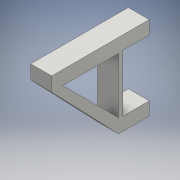
# Autodesk Inventor part: ServoSupport
Saved by Autodesk Inventor 2016 (Build 200138000, 138)
## iProperties
Created: 2016-04-17
Part Number: ServoSupport
Material: PC/ABS Plastic
Document SubType Name: Modeling
Designer: amenoni
Density: 0.357273 g/cm^3
Appearance: Smooth - White
Author: amenoni
Autodesk Inventor part; units mm, degrees
ref_plane "YZ Plane" through (0, 0, 0) normal (1, 0, 0) x (0, 1, 0)
ref_plane "XZ Plane" through (0, 0, 0) normal (0, 1, 0) x (-1, 0, 0)
ref_plane "XY Plane" through (0, 0, 0) normal (0, 0, 1) x (1, 0, 0)
sketch "Sketch1" plane through (0, 0, 0) normal (0, 1, 0) x (-1, 0, 0)
  line L0 (-7.5, -30) -> (7.5, -30)
  line L1 (7.5, -30) -> (7.5, 30)
  line L2 (7.5, 30) -> (-7.5, 30)
  line L3 (-7.5, 30) -> (-7.5, -30)
  line L4 (-7.5, -30) -> (7.5, 30) construction
  line L5 (7.5, -30) -> (-7.5, 30) construction
  point P0 (0, 0)
  dimension "d0" = 15
  dimension "d1" = 60
  constraints: 12 end point, 2 midpoint, 2 parallel, 1 horizontal, 1 perpendicular
  measures "d0" distance of L2.end L1.end
  measures "d1" distance of L1.end L0.end
extrude "Extrusion1" add sketch "Sketch1" along normal blind 3
sketch "Sketch2" plane through (0, 3, 0) normal (0, 1, 0) x (1, 0, 0)
  line L0 (-7.5, 30) -> (-7.5, -30) projected
  line L1 (7.5, 20.5) -> (-7.5, 20.5)
  line L2 (-7.5, 20.5) -> (-7.5, -20.5)
  line L3 (-7.5, -20.5) -> (7.5, -20.5)
  line L4 (7.5, -20.5) -> (7.5, 20.5)
  line L5 (7.5, 20.5) -> (-7.5, -20.5) construction
  line L6 (-7.5, 20.5) -> (7.5, -20.5) construction
  line L7 (7.5, -20.5) -> (-7.5, -20.5)
  line L8 (-7.5, -20.5) -> (-7.5, -30)
  line L9 (-7.5, -30) -> (7.5, -30)
  line L10 (7.5, -30) -> (7.5, -20.5)
  line L11 (7.5, 30) -> (-7.5, 30) projected
  line L12 (7.5, 20.5) -> (-7.5, 20.5)
  line L13 (-7.5, 20.5) -> (-7.5, 30)
  line L14 (-7.5, 30) -> (7.5, 30)
  line L15 (7.5, 30) -> (7.5, 20.5)
  point P0 (0, 0)
  dimension "d4" = 41
  constraints: 28 end point, 6 parallel, 3 horizontal, 3 perpendicular, 2 midpoint, 1 point on line
  measures "d4" distance of L2.end L1.end
extrude "Extrusion2" add sketch "Sketch2" along normal blind 19 contours L11 L15 L1 L0 | L3 L10 L9 L0
sketch "Sketch3" plane through (-7.5, 0, -30) normal (-1, 0, 0) x (0, 0, 1)
  line L0 (60, 0) -> (0, 0) projected
  line L1 (60, 0) -> (50, 0)
  line L2 (50, 0) -> (50, -48)
  line L3 (50, -48) -> (60, -48)
  line L4 (60, -48) -> (60, 0)
  point P0 (30, 0)
  dimension "d7" = 10
  dimension "d8" = 48
  constraints: 8 end point, 2 parallel, 1 horizontal, 1 perpendicular
  measures "d7" distance of L3.end L2.end
  measures "d8" distance of L2.end L1.end
extrude "Extrusion3" add sketch "Sketch3" against normal blind 15
sketch "Sketch4" plane through (-7.5, 0, -30) normal (-1, 0, 0) x (0, 0, 1)
  line L0 (0, 0) -> (0, 22) projected
  line L1 (0, 0) -> (10, 0)
  line L2 (50, 0) -> (0, 0) projected
  line L3 (10, 0) -> (50, -40)
  line L4 (50, -48) -> (50, 0) projected
  line L5 (10, 0) -> (66.5685, 0) construction
  line L6 (50, -40) -> (50, -48)
  line L7 (50, -48) -> (0, 0)
  point P0 (30, 0)
  dimension "d11" = 10
  dimension "d12" = 45
  constraints: 10 end point, 2 point on line, 1 collinear, 1 equal length, 1 horizontal
  measures "d11" distance of L0.start L1.end
  measures "d12" angle of L3 L5
extrude "Extrusion4" add sketch "Sketch4" against normal blind 15 contours L1 L3 L4 L7
body "Solid1"
